Autodesk Inventor part; units mm, degrees
(part 3 of 3)
sketch "Эскиз9" plane through (0, 0, 5) normal (0, 0, 1) x (1, 0, 0)
  circle A0 centre (1.2104, 5.1192) radius 2.5 projected
  circle A1 centre (1.2104, 5.1192) radius 12.2678
  line L0 (44.0249, 7.1187) -> (57, -5.9715) projected
  line L1 (57, -5.9715) -> (57, 20.778) projected
  line L2 (53, 20.778) -> (57, 20.778) projected
  line L3 (25.3405, 9.161) -> (53, 20.778) projected
  arc A2 (16.1963, 14.3431) -> (25.3405, 9.161) centre (40.8164, 47.1281) ccw projected
  arc A3 (16.1963, 14.3431) -> (-11.1891, 14.3431) centre (2.5036, -3.8906) ccw projected
  line L4 (-11.1891, 14.3431) -> (-11.0924, 14.1698) projected
  line L5 (-11.0924, 14.1698) -> (-10.8798, 13.8428) projected
  line L6 (-10.8798, 13.8428) -> (-10.6476, 13.5415) projected
  line L7 (-10.6476, 13.5415) -> (-10.3902, 13.2744) projected
  line L8 (-10.3902, 13.2744) -> (-10.0964, 13.0589) projected
  line L9 (-10.0964, 13.0589) -> (-9.8198, 12.8188) projected
  line L10 (-9.8198, 12.8188) -> (-9.6918, 12.6838) projected
  line L11 (-9.6918, 12.6838) -> (-9.5723, 12.5363) projected
  line L12 (-9.5723, 12.5363) -> (-9.4633, 12.3731) projected
  line L13 (-9.4633, 12.3731) -> (-9.3681, 12.1883) projected
  line L14 (-9.3681, 12.1883) -> (-9.3278, 12.0845) projected
  line L15 (-9.3278, 12.0845) -> (-9.2943, 11.9695) projected
  line L16 (-9.2943, 11.9695) -> (-9.2712, 11.8376) projected
  line L17 (-9.2712, 11.8376) -> (-9.2668, 11.6743) projected
  line L18 (-9.2668, 11.6743) -> (-9.3696, 11.329) projected
  line L19 (-9.3696, 11.329) -> (-9.7265, 10.6764) projected
  line L20 (-9.7265, 10.6764) -> (-10.0432, 10.0032) projected
  line L21 (-10.0432, 10.0032) -> (-10.2615, 9.7167) projected
  line L22 (-10.2615, 9.7167) -> (-10.3959, 9.6239) projected
  line L23 (-10.3959, 9.6239) -> (-10.5161, 9.5649) projected
  line L24 (-10.5161, 9.5649) -> (-10.6287, 9.5241) projected
  line L25 (-10.6287, 9.5241) -> (-10.7364, 9.4955) projected
  line L26 (-10.7364, 9.4955) -> (-10.9417, 9.4634) projected
  line L27 (-10.9417, 9.4634) -> (-11.1379, 9.4552) projected
  line L28 (-11.1379, 9.4552) -> (-11.3274, 9.4648) projected
  line L29 (-11.3274, 9.4648) -> (-11.5119, 9.4885) projected
  line L30 (-11.5119, 9.4885) -> (-11.8689, 9.5704) projected
  line L31 (-11.8689, 9.5704) -> (-12.2162, 9.6807) projected
  line L32 (-12.2162, 9.6807) -> (-12.5837, 9.731) projected
  line L33 (-12.5837, 9.731) -> (-12.964, 9.741) projected
  line L34 (-12.964, 9.741) -> (-13.3534, 9.7199) projected
  line L35 (-13.3534, 9.7199) -> (-13.7498, 9.6714) projected
  line L36 (-13.7498, 9.6714) -> (-14.1519, 9.5976) projected
  line L37 (-14.1519, 9.5976) -> (-14.5586, 9.4998) projected
  line L38 (-14.5586, 9.4998) -> (-14.9687, 9.3787) projected
  line L39 (-14.9687, 9.3787) -> (-15.3815, 9.2349) projected
  line L40 (-15.3815, 9.2349) -> (-15.796, 9.069) projected
  line L41 (-15.796, 9.069) -> (-16.1075, 8.9301) projected
  line L42 (-16.1075, 8.9301) -> (-16.4414, 6.8067) projected
  line L43 (-16.4414, 6.8067) -> (-16.1875, 6.579) projected
  line L44 (-16.1875, 6.579) -> (-15.8439, 6.2938) projected
  line L45 (-15.8439, 6.2938) -> (-15.4952, 6.0303) projected
  line L46 (-15.4952, 6.0303) -> (-15.142, 5.7892) projected
  line L47 (-15.142, 5.7892) -> (-14.785, 5.5713) projected
  line L48 (-14.785, 5.5713) -> (-14.425, 5.3776) projected
  line L49 (-14.425, 5.3776) -> (-14.0625, 5.2099) projected
  line L50 (-14.0625, 5.2099) -> (-13.6984, 5.0703) projected
  line L51 (-13.6984, 5.0703) -> (-13.3334, 4.963) projected
  line L52 (-13.3334, 4.963) -> (-12.9682, 4.8982) projected
  line L53 (-12.9682, 4.8982) -> (-12.6038, 4.8965) projected
  line L54 (-12.6038, 4.8965) -> (-12.2389, 4.8649) projected
  line L55 (-12.2389, 4.8649) -> (-12.056, 4.8309) projected
  line L56 (-12.056, 4.8309) -> (-11.8727, 4.7818) projected
  line L57 (-11.8727, 4.7818) -> (-11.6885, 4.7139) projected
  line L58 (-11.6885, 4.7139) -> (-11.5029, 4.6203) projected
  line L59 (-11.5029, 4.6203) -> (-11.4093, 4.56) projected
  line L60 (-11.4093, 4.56) -> (-11.3146, 4.4866) projected
  line L61 (-11.3146, 4.4866) -> (-11.2183, 4.3936) projected
  line L62 (-11.2183, 4.3936) -> (-11.1188, 4.264) projected
  line L63 (-11.1188, 4.264) -> (-10.999, 3.9243) projected
  line L64 (-10.999, 3.9243) -> (-10.9042, 3.1865) projected
  line L65 (-10.9042, 3.1865) -> (-10.7647, 2.4558) projected
  line L66 (-10.7647, 2.4558) -> (-10.7729, 2.0956) projected
  line L67 (-10.7729, 2.0956) -> (-10.8272, 1.9416) projected
  line L68 (-10.8272, 1.9416) -> (-10.8897, 1.8232) projected
  line L69 (-10.8897, 1.8232) -> (-10.9568, 1.724) projected
  line L70 (-10.9568, 1.724) -> (-11.0271, 1.6375) projected
  line L71 (-11.0271, 1.6375) -> (-11.1743, 1.4909) projected
  line L72 (-11.1743, 1.4909) -> (-11.3282, 1.369) projected
  line L73 (-11.3282, 1.369) -> (-11.4872, 1.2653) projected
  line L74 (-11.4872, 1.2653) -> (-11.6504, 1.1761) projected
  line L75 (-11.6504, 1.1761) -> (-11.9874, 1.0325) projected
  line L76 (-11.9874, 1.0325) -> (-12.3332, 0.9175) projected
  line L77 (-12.3332, 0.9175) -> (-12.66, 0.7423) projected
  line L78 (-12.66, 0.7423) -> (-12.9736, 0.5268) projected
  line L79 (-12.9736, 0.5268) -> (-13.2762, 0.2808) projected
  line L80 (-13.2762, 0.2808) -> (-13.5684, 0.0086) projected
  line L81 (-13.5684, 0.0086) -> (-13.8504, -0.2874) projected
  line L82 (-13.8504, -0.2874) -> (-14.1218, -0.6056) projected
  line L83 (-14.1218, -0.6056) -> (-14.3824, -0.9447) projected
  line L84 (-14.3824, -0.9447) -> (-14.6319, -1.3036) projected
  line L85 (-14.6319, -1.3036) -> (-14.8697, -1.6815) projected
  line L86 (-14.8697, -1.6815) -> (-15.0401, -1.9769) projected
  line L87 (-15.0401, -1.9769) -> (-14.0621, -3.891) projected
  line L88 (-14.0621, -3.891) -> (-13.7228, -3.9261) projected
  line L89 (-13.7228, -3.9261) -> (-13.2773, -3.9548) projected
  line L90 (-13.2773, -3.9548) -> (-12.8403, -3.963) projected
  line L91 (-12.8403, -3.963) -> (-12.4128, -3.9505) projected
  line L92 (-12.4128, -3.9505) -> (-11.9959, -3.917) projected
  line L93 (-11.9959, -3.917) -> (-11.5908, -3.862) projected
  line L94 (-11.5908, -3.862) -> (-11.199, -3.7847) projected
  line L95 (-11.199, -3.7847) -> (-10.8224, -3.6836) projected
  line L96 (-10.8224, -3.6836) -> (-10.464, -3.5558) projected
  line L97 (-10.464, -3.5558) -> (-10.1304, -3.3936) projected
  line L98 (-10.1304, -3.3936) -> (-9.8347, -3.1808) projected
  line L99 (-9.8347, -3.1808) -> (-9.5209, -2.9918) projected
  line L100 (-9.5209, -2.9918) -> (-9.353, -2.9118) projected
  line L101 (-9.353, -2.9118) -> (-9.1758, -2.8438) projected
  line L102 (-9.1758, -2.8438) -> (-8.9868, -2.7905) projected
  line L103 (-8.9868, -2.7905) -> (-8.7817, -2.7571) projected
  line L104 (-8.7817, -2.7571) -> (-8.6705, -2.7509) projected
  line L105 (-8.6705, -2.7509) -> (-8.5508, -2.7546) projected
  line L106 (-8.5508, -2.7546) -> (-8.4182, -2.7733) projected
  line L107 (-8.4182, -2.7733) -> (-8.2615, -2.8196) projected
  line L108 (-8.2615, -2.8196) -> (-7.9649, -3.024) projected
  line L109 (-7.9649, -3.024) -> (-7.4545, -3.5652) projected
  line L110 (-7.4545, -3.5652) -> (-6.9122, -4.0744) projected
  line L111 (-6.9122, -4.0744) -> (-6.7071, -4.3705) projected
  line L112 (-6.7071, -4.3705) -> (-6.6604, -4.5271) projected
  line L113 (-6.6604, -4.5271) -> (-6.6415, -4.6596) projected
  line L114 (-6.6415, -4.6596) -> (-6.6374, -4.7793) projected
  line L115 (-6.6374, -4.7793) -> (-6.6435, -4.8906) projected
  line L116 (-6.6435, -4.8906) -> (-6.6764, -5.0958) projected
  line L117 (-6.6764, -5.0958) -> (-6.7292, -5.2848) projected
  line L118 (-6.7292, -5.2848) -> (-6.7969, -5.4622) projected
  line L119 (-6.7969, -5.4622) -> (-6.8765, -5.6303) projected
  line L120 (-6.8765, -5.6303) -> (-7.0647, -5.9445) projected
  line L121 (-7.0647, -5.9445) -> (-7.2769, -6.2407) projected
  line L122 (-7.2769, -6.2407) -> (-7.4384, -6.5746) projected
  line L123 (-7.4384, -6.5746) -> (-7.5654, -6.9333) projected
  line L124 (-7.5654, -6.9333) -> (-7.6656, -7.3102) projected
  line L125 (-7.6656, -7.3102) -> (-7.742, -7.7022) projected
  line L126 (-7.742, -7.7022) -> (-7.7961, -8.1074) projected
  line L127 (-7.7961, -8.1074) -> (-7.8287, -8.5243) projected
  line L128 (-7.8287, -8.5243) -> (-7.8403, -8.9518) projected
  line L129 (-7.8403, -8.9518) -> (-7.8311, -9.3888) projected
  line L130 (-7.8311, -9.3888) -> (-7.8013, -9.8343) projected
  line L131 (-7.8013, -9.8343) -> (-7.7656, -10.1735) projected
  line L132 (-7.7656, -10.1735) -> (-5.8492, -11.1472) projected
  line L133 (-5.8492, -11.1472) -> (-5.5542, -10.9761) projected
  line L134 (-5.5542, -10.9761) -> (-5.1768, -10.7375) projected
  line L135 (-5.1768, -10.7375) -> (-4.8185, -10.4872) projected
  line L136 (-4.8185, -10.4872) -> (-4.48, -10.2258) projected
  line L137 (-4.48, -10.2258) -> (-4.1624, -9.9537) projected
  line L138 (-4.1624, -9.9537) -> (-3.867, -9.6711) projected
  line L139 (-3.867, -9.6711) -> (-3.5955, -9.3782) projected
  line L140 (-3.5955, -9.3782) -> (-3.3502, -9.0751) projected
  line L141 (-3.3502, -9.0751) -> (-3.1354, -8.7611) projected
  line L142 (-3.1354, -8.7611) -> (-2.9609, -8.4338) projected
  line L143 (-2.9609, -8.4338) -> (-2.8467, -8.0877) projected
  line L144 (-2.8467, -8.0877) -> (-2.7039, -7.7505) projected
  line L145 (-2.7039, -7.7505) -> (-2.615, -7.5871) projected
  line L146 (-2.615, -7.5871) -> (-2.5117, -7.4278) projected
  line L147 (-2.5117, -7.4278) -> (-2.3901, -7.2737) projected
  line L148 (-2.3901, -7.2737) -> (-2.2438, -7.1261) projected
  line L149 (-2.2438, -7.1261) -> (-2.1575, -7.0556) projected
  line L150 (-2.1575, -7.0556) -> (-2.0585, -6.9883) projected
  line L151 (-2.0585, -6.9883) -> (-1.9402, -6.9255) projected
  line L152 (-1.9402, -6.9255) -> (-1.7863, -6.8709) projected
  line L153 (-1.7863, -6.8709) -> (-1.4262, -6.8619) projected
  line L154 (-1.4262, -6.8619) -> (-0.6951, -6.9997) projected
  line L155 (-0.6951, -6.9997) -> (0.0429, -7.0929) projected
  line L156 (0.0429, -7.0929) -> (0.3829, -7.2119) projected
  line L157 (0.3829, -7.2119) -> (0.5127, -7.3112) projected
  line L158 (0.5127, -7.3112) -> (0.6059, -7.4072) projected
  line L159 (0.6059, -7.4072) -> (0.6795, -7.5017) projected
  line L160 (0.6795, -7.5017) -> (0.74, -7.5953) projected
  line L161 (0.74, -7.5953) -> (0.834, -7.7806) projected
  line L162 (0.834, -7.7806) -> (0.9024, -7.9646) projected
  line L163 (0.9024, -7.9646) -> (0.9519, -8.1479) projected
  line L164 (0.9519, -8.1479) -> (0.9863, -8.3307) projected
  line L165 (0.9863, -8.3307) -> (1.0187, -8.6955) projected
  line L166 (1.0187, -8.6955) -> (1.0212, -9.0599) projected
  line L167 (1.0212, -9.0599) -> (1.0869, -9.4249) projected
  line L168 (1.0869, -9.4249) -> (1.1949, -9.7897) projected
  line L169 (1.1949, -9.7897) -> (1.3353, -10.1535) projected
  line L170 (1.3353, -10.1535) -> (1.5039, -10.5156) projected
  line L171 (1.5039, -10.5156) -> (1.6983, -10.8752) projected
  line L172 (1.6983, -10.8752) -> (1.9171, -11.2317) projected
  line L173 (1.9171, -11.2317) -> (2.159, -11.5843) projected
  line L174 (2.159, -11.5843) -> (2.4233, -11.9325) projected
  line L175 (2.4233, -11.9325) -> (2.7092, -12.2754) projected
  line L176 (2.7092, -12.2754) -> (2.9375, -12.5288) projected
  line L177 (2.9375, -12.5288) -> (5.0602, -12.1901) projected
  line L178 (5.0602, -12.1901) -> (5.1983, -11.8783) projected
  line L179 (5.1983, -11.8783) -> (5.3633, -11.4634) projected
  line L180 (5.3633, -11.4634) -> (5.5062, -11.0504) projected
  line L181 (5.5062, -11.0504) -> (5.6263, -10.6399) projected
  line L182 (5.6263, -10.6399) -> (5.7233, -10.2331) projected
  line L183 (5.7233, -10.2331) -> (5.7962, -9.8308) projected
  line L184 (5.7962, -9.8308) -> (5.8437, -9.4343) projected
  line L185 (5.8437, -9.4343) -> (5.864, -9.0449) projected
  line L186 (5.864, -9.0449) -> (5.8532, -8.6645) projected
  line L187 (5.8532, -8.6645) -> (5.802, -8.2972) projected
  line L188 (5.802, -8.2972) -> (5.691, -7.9502) projected
  line L189 (5.691, -7.9502) -> (5.6083, -7.5933) projected
  line L190 (5.6083, -7.5933) -> (5.5841, -7.4089) projected
  line L191 (5.5841, -7.4089) -> (5.5741, -7.2193) projected
  line L192 (5.5741, -7.2193) -> (5.5818, -7.0232) projected
  line L193 (5.5818, -7.0232) -> (5.6135, -6.8178) projected
  line L194 (5.6135, -6.8178) -> (5.6419, -6.7101) projected
  line L195 (5.6419, -6.7101) -> (5.6824, -6.5974) projected
  line L196 (5.6824, -6.5974) -> (5.7412, -6.4771) projected
  line L197 (5.7412, -6.4771) -> (5.8336, -6.3424) projected
  line L198 (5.8336, -6.3424) -> (6.1197, -6.1235) projected
  line L199 (6.1197, -6.1235) -> (6.7921, -5.8052) projected
  line L200 (6.7921, -5.8052) -> (7.444, -5.4468) projected
  line L201 (7.444, -5.4468) -> (7.789, -5.3433) projected
  line L202 (7.789, -5.3433) -> (7.9523, -5.3473) projected
  line L203 (7.9523, -5.3473) -> (8.0842, -5.3702) projected
  line L204 (8.0842, -5.3702) -> (25.3405, 4.0009) projected
  line L205 (40.9018, 10.5367) -> (25.3405, 4.0009) projected
  line L206 (40.9018, 10.5367) -> (44.0249, 7.1187) projected
  circle A4 centre (1.2104, 5.1192) radius 2.5 projected
  circle A5 centre (4.7663, 12.2855) radius 1.6 projected
  circle A6 centre (-5.9559, 8.675) radius 1.6 projected
  circle A7 centre (-2.3455, -2.0471) radius 1.6 projected
  circle A8 centre (8.3767, 1.5633) radius 1.6 projected
  point P0 (0, 0)
  point P1 (-10.9042, 3.1865)
  constraints: 1 coincident, 3 other
extrude "Выдавливание9" cut sketch "Эскиз9" against normal through all contours A1 L18 L17 L16 L15 L14 L13 L12 L11 L10 L9 L8 L7 L6 L5 L4 A3 A2 L3 L2 L1 L0 L206 L205 L204 L203 L202 L201
sketch "Эскиз16" plane through (0, 0, 5) normal (0, 0, 1) x (1, 0, 0)
  line L0 (79.8483, -54.0962) -> (75.1417, -35.0972) projected
  line L1 (75.1417, -35.0972) -> (67.3253, -3.5443)
  line L2 (79.8483, -54.0962) -> (83.7309, -53.1344)
  line L3 (83.7309, -53.1344) -> (70.5682, 0)
  arc A0 (7.444, -5.4468) -> (-9.3696, 11.329) centre (1.2104, 5.1192) ccw projected
  line L4 (12, -0.7188) -> (13.7212, 2.8919)
  line L5 (12.8606, 8.9625) -> (70.5682, 0)
  line L6 (13.4745, 4.8192) -> (67.3253, -3.5443)
  point P0 (0, 0)
  dimension "d45" = 4
  dimension "d46" = 4
  constraints: 12 end point, 3 point on circle, 2 parallel, 1 perpendicular, 1 other
  measures "d45" distance of L0.start L2.end
  measures "d46" distance of L4.start L4.end
extrude "Выдавливание15" add sketch "Эскиз16" against normal up to surface (5 mm away) contours L0 L1 L6 A0 L5 L3 L2
sketch "Эскиз17" plane through (0, 0, 5) normal (0, 0, 1) x (1, 0, 0)
  point P0 (0, 0)
